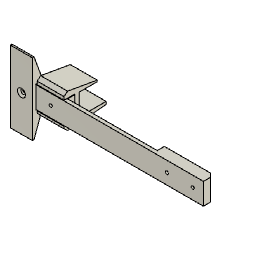
スマホ台 v1 (Autodesk Fusion 360 design; units mm, degrees)
Autodesk Fusion 360 part; units mm, degrees
sketch "スケッチ1" plane through (0, 0, 0) normal (0, 1, 0) x (1, 0, 0)
  line L0 (45, 6) -> (-45, 6)
  line L1 (-45, 6) -> (-45, -6)
  line L2 (-45, -6) -> (45, -6)
  line L3 (45, -6) -> (45, 6)
  line L4 (45, 6) -> (-45, -6) construction
  line L5 (-45, 6) -> (45, -6) construction
  line L6 (-45, -6) -> (-45, -9)
  line L7 (-45, -9) -> (-30, -9)
  line L8 (-30, -9) -> (-30, -6)
  line L9 (-53, 0) -> (-70, 0)
  line L10 (-45, 6) -> (-45, 9)
  line L11 (-45, 9) -> (-30, 9)
  line L12 (-30, 9) -> (-30, 6)
  line L13 (0, -19) -> (0, -11)
  line L14 (45, -9) -> (30, -9)
  line L15 (45, -6) -> (45, -9)
  line L16 (30, -9) -> (30, -6)
  line L17 (45, 6) -> (45, 9)
  line L18 (30, 9) -> (30, 6)
  line L19 (45, 9) -> (30, 9)
  line L20 (-30, -6) -> (-30, 6)
  line L21 (30, -6) -> (30, 6)
  dimension "d1" = 90
  dimension "d2" = 12
  dimension "d3" = 3
  constraint horizontal L0
  constraint perpendicular L0 L1
  constraint parallel L0 L2
  constraint parallel L1 L3
  constraint coincident L4 origin
  constraint coincident L5 origin
  constraint perpendicular L2 L6
  constraint perpendicular L6 L7
  constraint coincident L2 L8.end
  constraint perpendicular L2 L8
  constraint perpendicular L1 L9
  constraint symmetric L1.end L9 L0.end
  constraint symmetric L6.end L9 L10.end
  constraint symmetric L7.end L9 L11.end
  constraint symmetric L8.end L9 L12.end
  constraint vertical L13
  constraint symmetric L1.end L13 L2.end
  constraint symmetric L6.end L13 L14.start
  constraint symmetric L7.end L13 L14.end
  constraint symmetric L8.end L13 L16.end
  constraint symmetric L0.end L13 L0.start
  constraint symmetric L10.end L13 L17.end
  constraint symmetric L11.end L13 L18.start
  constraint symmetric L12.end L13 L18.end
  measures "d1" distance of L1.end L2.end
  measures "d2" distance of L0.end L1.end
  measures "d3" distance of L1.end L6.end
extrude "押し出し1" add sketch "スケッチ1" along normal blind 2 contours L0 L2 L3 L21 | L0 L2 L20 L21 | L0 L1 L2 L20 makes body 1
extrude "押し出し2" add sketch "スケッチ1" along normal blind 2.5 from surface at 2 separate body contours L0 L1 L2 L20 | L0 L10 L11 L12 | L2 L6 L7 L8 makes body 2
extrude "押し出し3" add sketch "スケッチ1" along normal blind 15 from surface at 4.5 separate body contours L0 L10 L11 L12 | L2 L6 L7 L8 makes body 3 at (-35, 9.5, -6) makes body 4 at (-40, 9.5, 9)
move_face "面を移動1" by (0, -7, 0) 1 faces at (-40, 19.5, 7) on bodies 4
move_face "面を移動2" by (0, 2, 0) 1 faces at (-35, 12.5, 8) on bodies 4
combine "結合1" operation add target body 3 tool bodies 4 2
move_body "移動1" bodies 3 to x (1, 0, 0) y (0, 1, 0) z (0, 0, 1) at (0, 4, 0)
extrude "押し出し4" add sketch "スケッチ1" along normal blind 6 separate body contours L0 L1 L2 L20 makes body 5
combine "結合2" operation add target body 5 tool bodies 1
sketch "スケッチ2" plane through (0, 0, 0) normal (0, 1, 0) x (1, 0, 0)
  line L0 (-29.2493, 6) -> (-17, 6)
  line L1 (-17, 6) -> (-17, -20)
  line L2 (-17, -20) -> (-29.2493, -20)
  line L3 (-29.2493, -20) -> (-29.2493, 6)
  line L4 (45, 6) -> (-45, 6)
  line L5 (-29.2493, -6) -> (-17, -6)
  line L6 (-17, -6) -> (-17, -6)
  line L7 (-17, -6) -> (-29.2493, -6)
  line L8 (-29.2493, -6) -> (-29.2493, -6)
  line L9 (-29.2493, 0) -> (-17, 0)
  line L10 (-29.2493, 20) -> (-29.2493, -6)
  line L11 (-17, -6) -> (-17, 20)
  line L12 (-17, 20) -> (-29.2493, 20)
  constraint horizontal L0
  constraint vertical L1
  constraint horizontal L2
  constraint vertical L3
  constraint coincident L0.start L4
  constraint horizontal L5
  constraint horizontal L7
  constraint coincident L1 L5.end
  constraint coincident L3 L5.start
  constraint coincident L3 L9.start
  constraint coincident L1 L9.end
  constraint perpendicular L1 L9
  constraint symmetric L0.start L9 L5.start
  constraint symmetric L0.end L9 L5.end
  constraint symmetric L1.end L9 L11.end
  constraint symmetric L2.end L9 L10.start
extrude "押し出し5" add sketch "スケッチ2" along normal blind 6 separate body contours L0 L4 L10 L11 L12 | L1 L2 L3 L5 L7 makes body 6 at (-21.0831, 0, -15.3333) makes body 7 at (-21.0831, 0, 15.3333)
move_face "面を移動3" to x (1, 0, 0) y (0, 0.939693, -0.34202) z (0, 0.34202, 0.939693) at (0, 2.414, 1.6903) 1 faces at (-21.0831, 6, -15.3333) on bodies 6
move_face "面を移動4" to x (1, 0, 0) y (0, 0.939693, 0.34202) z (0, -0.34202, 0.939693) at (0, 2.414, -1.6903) 1 faces at (-21.0831, 6, 15.3333) on bodies 7
move_body "移動2" bodies 7 6 to x (1, 0, 0) y (0, 1, 0) z (0, 0, 1) at (0, -2, 0)
move_face "面を移動5" to x (1, 0, 0) y (0, 0.984808, -0.173648) z (0, 0.173648, 0.984808) at (0, -1.4717, 1.1786) 1 faces at (-40, 10.1667, 9) on bodies 3
move_face "面を移動6" to x (1, 0, 0) y (0, 0.996195, 0.087156) z (0, -0.087156, 0.996195) at (0, -0.7616, -0.5572) 1 faces at (-40, 11.8333, -9) on bodies 3
sketch "スケッチ3" plane through (0, 0, -6) normal (0, 0, 1) x (-1, 0, 0)
  line L0 (29.2493, 2) -> (17, 2)
  line L1 (17, 2) -> (17, -4)
  line L2 (17, -4) -> (29.2493, -4)
  line L3 (29.2493, -4) -> (29.2493, 2)
  line L4 (17, 2) -> (29.2493, 2)
  line L5 (29.2493, 2) -> (29.2493, 0)
  line L6 (29.2493, 0) -> (17, 0)
  line L7 (17, 0) -> (17, 2)
  constraint horizontal L4
  constraint vertical L5
  constraint horizontal L6
  constraint vertical L7
  constraint coincident L3 L5.end
  constraint coincident L0.end L1.start
extrude "押し出し6" add sketch "スケッチ3" along normal blind 12 separate body contours L0 L1 L3 L4 L5 L6 L7 makes body 8
combine "結合3" operation add target body 6 tool bodies 8 7
move_body "移動3" bodies 6 to x (1, 0, 0) y (0, 1, 0) z (0, 0, 1) at (-5, 0, 0)
move_face "面を移動7" by (9, 0, 0) 1 faces at (-30, 3.3333, 2) on bodies 5
move_body "移動4" bodies 6 to x (1, 0, 0) y (0, 1, 0) z (0, 0, 1) at (5, 0, 0)
move_face "面を移動8" by (5, 0, 0) 1 faces at (-21, 3.3333, 2) on bodies 5
split "分割1" by plane through (-30, 8.5, -6) normal (0, 0, 1) and through (-45, 8.5, 6) normal (0, 0, -1) bodies 3 makes body 9 at (-40, 10.1667, 8.2653) makes body 10 at (-35, 8.5, 2)
move_face "面を移動9" by (0, -6, 0) 2 faces at (-35, 6, -7) (-35, 6, 8) on bodies 3 9
combine "結合4" operation add target body 3 tool bodies 10 9
split "分割2" by plane through (0, 0, 0) normal (1, 0, 0) bodies 5 makes body 11 at (15, 0, 2)
delete_body "RemoveBody1" bodies 11
sketch "スケッチ4" plane through (0, -2, 0) normal (0, -1, 0) x (1, 0, 0)
  line L0 (-17, -20) -> (-17, 20)
  line L1 (-17, 20) -> (-29.2493, 20)
  line L2 (-29.2493, 20) -> (-29.2493, -20)
  line L3 (-29.2493, -20) -> (-17, -20)
  circle A0 centre (-23.1246, 0) radius 6.1246
  circle A1 centre (-23.1246, 0) radius 1.25
  dimension "d21" = 2.5
  constraint tangent L2 A0
  constraint concentric A0 A1
  measures "d21" diameter of A1
extrude "押し出し7" cut sketch "スケッチ4" against normal blind 9 contours A1 bodies 5 6
chamfer "面取り1" distance 1 angle 45 1 edges at (-24.2901, -2, 0.452) on bodies 6
move_face "面をオフセット1" offset 0.4 1 faces at (-21.8809, 2, -0.1245) on bodies 5
move_face "面を移動10" to x (0.766044, 0.642788, 0) y (-0.642788, 0.766044, 0) z (0, 0, 1) at (-1.5917, 11.2525, 0) 1 faces at (-16, 4.6667, -2) on bodies 5
sketch "スケッチ5" plane through (0, 8.5, 0) normal (0, 1, 0) x (-1, 0, 0)
  line L0 (30, -6) -> (45, -6)
  line L1 (45, -6) -> (45, 6)
  line L2 (45, 6) -> (30, 6)
  line L3 (30, 6) -> (30, -6)
  circle A0 centre (37.5, 0) radius 6
  circle A1 centre (37.5, 0) radius 1.25
  dimension "d26" = 2.5
  constraint tangent L0 A0
  constraint concentric A0 A1
  measures "d26" diameter of A1
extrude "押し出し8" cut sketch "スケッチ5" against normal blind 18 contours A1 bodies 3 5
chamfer "面取り2" distance 1 angle 45 1 edges at (-36.3346, 8.5, 0.452) on bodies 3
move_face "面をオフセット2" offset 0.4 1 faces at (-38.7438, 4, -0.1245) on bodies 5
sketch "スケッチ6" plane through (0, 2, 0) normal (0, 1, 0) x (-1, 0, 0)
  line L0 (0, 6) -> (0, -6)
  line L1 (0, -6) -> (14.7144, -6)
  line L2 (14.7144, -6) -> (14.7144, 6)
  line L3 (14.7144, 6) -> (0, 6)
  line L4 (18, -1) -> (-3.2856, -1)
  line L5 (-3.2856, -1) -> (-3.2856, 1)
  line L6 (-3.2856, 1) -> (18, 1)
  line L7 (18, 1) -> (18, -1)
  line L8 (18, -1) -> (-3.2856, 1) construction
  line L9 (-3.2856, -1) -> (18, 1) construction
  point P0 (7.3572, 0)
  constraint horizontal L4
  constraint perpendicular L4 L5
  constraint parallel L4 L6
  constraint parallel L5 L7
  constraint coincident L8 P0
  constraint coincident L9 P0
extrude "押し出し9" add sketch "スケッチ6" along normal blind 3 separate body contours L0 L2 L4 L6 | L2 L4 L6 L7 makes body 12
combine "結合5" operation add target body 12 tool bodies 5
move_face "面を移動11" by (0, 0, 0.3) 1 faces at (-25.1662, 2.6667, 6) on bodies 6
move_face "面を移動12" by (0, 0, -0.3) 1 faces at (-21.0831, 1.3333, -6) on bodies 6
move_face "面を移動13" by (0, 0, 0.3) 1 faces at (-40, 2, 6) on bodies 3
move_face "面を移動14" by (0, 0, -0.3) 1 faces at (-35, 2, -6) on bodies 3
chamfer "面取り3" distance 2 angle 45 1 edges at (-37.5, 0, -9.5249) on bodies 3
chamfer "面取り4" distance 2 angle 45 1 edges at (-37.5, 0, 10.058) on bodies 3
sketch "スケッチ7" plane through (0, 6, 0) normal (0, -1, 0) x (1, 0, 0)
  circle A0 centre (-37.5, 0) radius 1.25
  line L0 (-30, 6.3) -> (-45, 6.3)
  line L1 (-45, 6.3) -> (-45, -6.3)
  line L2 (-45, -6.3) -> (-30, -6.3)
  line L3 (-30, -6.3) -> (-30, 6.3)
  line L4 (-39.5, 0) -> (-38.2813, -0.9758)
  line L5 (-39.5, 0) -> (-38.8906, 0)
  line L6 (-39.5, 0) -> (-38.2813, 0.9758)
  constraint coincident A0 L4.end
  constraint tangent A0 L4
  constraint horizontal L5
  constraint symmetric L4.start L5 L6.start
  constraint symmetric L4.end L5 L6.end
extrude "押し出し10" cut sketch "スケッチ7" against normal blind 2 contours A0 L4 L6 bodies 3
delete_face "面を削除1" 1 faces at (-39.3329, 8, 0.0234) on bodies 3
move_body "移動5" bodies 3 to x (1, 0, 0) y (0, 1, 0) z (0, 0, 1) at (14.3, 0, 0)
move_body "移動6" bodies 6 to x (1, 0, 0) y (0, 1, 0) z (0, 0, 1) at (-14.35, 0, 0)
move_face "面を移動15" by (1.5, 0, 0) 1 faces at (-45, 2, 2) on bodies 12
move_face "面を移動16" to x (0.773916, -0.633173, -0.012082) y (0.63325, 0.773517, 0.025792) z (-0.006985, -0.027611, 0.999594) at (-5.1176, -8.9665, -0.2344) 1 faces at (-16.6723, 4.3333, 4.3333) on bodies 12
split "分割3" by plane through (-15.7, 8.5, -9) normal (1, 0, 0) bodies 12 makes body 13 at (-10.4667, 0, -2)
delete_face "面を削除2" 1 faces at (-15.3002, 4.3333, 4.3333) on bodies 13
combine "結合6" operation add target body 13 tool bodies 12
move_face "面を移動17" by (10, 0, 0) 1 faces at (0, 0.6667, 0.3333) on bodies 13
move_face "面を移動18" by (-0.7, 0, 0) 1 faces at (10, 0.6667, 0.3333) on bodies 13
chamfer "面取り5" distance 2 angle 45 1 edges at (-43.5, 6, 0) on bodies 13
mirror "ミラー1" about plane through (9.3, 2, 1) normal (1, 0, 0) of bodies 13 merged
named bodies: "003", "002", "001"
